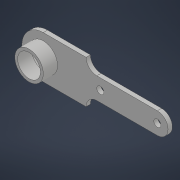
# Autodesk Inventor part: Shared Sketch
Saved by Autodesk Inventor 2022.4 (Build 264492000, 492)
## iProperties
Created: 2015-01-20
Part Number: Shared Sketch
Material: Generic
Document SubType Name: Modeling
Designer: jmacmillan
Density: 1 g/cm^3
Appearance: Default
Mass: 52.0264 g
Surface Area: 235.409 cm^2
Volume: 52.0264 cm^3
Author: jmacmillan
Autodesk Inventor part; units mm, degrees
ref_plane "YZ Plane" through (0, 0, 0) normal (1, 0, 0) x (0, 1, 0)
ref_plane "XZ Plane" through (0, 0, 0) normal (0, 1, 0) x (-1, 0, 0)
ref_plane "XY Plane" through (0, 0, 0) normal (0, 0, 1) x (1, 0, 0)
sketch "Sketch1" plane through (0, 0, 0) normal (0, 1, 0) x (-1, 0, 0)
  line L0 (0, -42) -> (0, 42) projected
  line L1 (-216, 0) -> (71, 0) projected
  circle A0 centre (0, 0) radius 16
  circle A1 centre (0, 0) radius 20
  arc A2 (0, -30) -> (0, 30) centre (0, 0) ccw
  line L2 (0, 30) -> (-60, 30)
  arc A3 (-75, 15) -> (-60, 30) centre (-75, 30) ccw
  line L3 (-75, 15) -> (-160, 15)
  arc A4 (-160, 15) -> (-160, -15) centre (-160, 0) ccw
  line L4 (0, -30) -> (-60, -30)
  arc A5 (-60, -30) -> (-75, -15) centre (-75, -30) ccw
  line L5 (-75, -15) -> (-160, -15)
  circle A6 centre (-160, 0) radius 5
  circle A7 centre (-80, 0) radius 5
  point P0 (0, 20)
  point P1 (0, 16)
  point P2 (-16, 0)
  point P3 (-20, 0)
  dimension "d0" = 30
  dimension "d1" = 40
  dimension "d2" = 4
  dimension "d3" = 10
  dimension "d4" = 80
  dimension "d5" = 60
  dimension "d6" = 160
  dimension "d8" = 15
  dimension "d10" = 15
  constraints: 8 centre point, 8 end point, 8 point on circle, 4 coincident, 4 symmetric about line, 4 tangent, 2 horizontal, 1 equal radius, 1 horizontal alignment, 1 point on line, 1 other
  measures "d0" radius of A2
  measures "d1" diameter of A1
  measures "d2" radial gap between concentric circles of A1 A0
  measures "d3" diameter of A6
  measures "d4" distance from line of A7.centre L0
  measures "d5" distance of L2.start L2.end
  measures "d6" distance from line of A4.centre L0
  measures "d8" radius of A4
  measures "d10" radius of A3
extrude "Extrusion1" add sketch "Sketch1" along normal blind 6 contours L4 A5 L5 A4 L1 A6 A7 A1 L0 | L0 A1 L1 A2 | A1 L1 A0 L0 | L0 A0 L1 A1 | L1 A1 L0 A2 | A1 L0 A0 L1 | L1 A7 A6 A4 L3 A3 L2 L0 A1 | L1 A0 L0 A1
extrude "Extrusion2" add sketch "Sketch1" against normal blind 20 contours A1 L1 A0 L0 | L0 A0 L1 A1 | A1 L0 A0 L1 | L1 A0 L0 A1
extrude "Extrusion3" cut sketch "Sketch1" along normal through all contours A1 L1 A0 L0 | L0 A0 L1 A1 | L1 A0 L0 A1 | L1 A0 L0 picked at (-18.3658, -2.6703) picked at (17.7056, -5.5628) picked at (18.4995, 1.4835) picked at (-10.5329, 1.1868)
body "Solid1"
